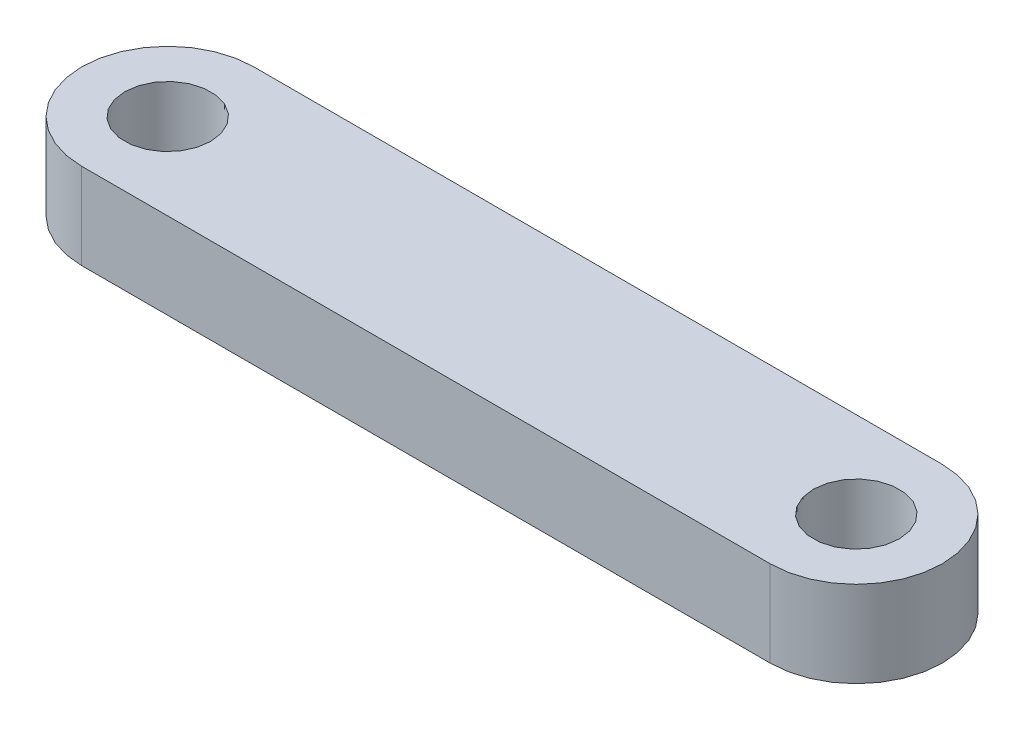
# Autodesk Inventor part: config_arm
Saved by Autodesk Inventor 2021 (Build 250183000, 183)
## iProperties
Created: 2020-12-29
Part Number: config_arm
Material: ABS Plastic
Document SubType Name: Modeling
Designer: Tomasz
Density: 1.06 g/cm^3
Appearance: Smooth - Black
Author: Tomasz
Autodesk Inventor part; units mm, degrees
ref_plane "YZ Plane" through (0, 0, 0) normal (1, 0, 0) x (0, 1, 0)
ref_plane "XZ Plane" through (0, 0, 0) normal (0, 1, 0) x (-1, 0, 0)
ref_plane "XY Plane" through (0, 0, 0) normal (0, 0, 1) x (1, 0, 0)
sketch "Sketch1" plane through (0, 0, 0) normal (0, 1, 0) x (-1, 0, 0)
  line L0 (-4, 0) -> (-36, 0)
  line L1 (-40, -4) -> (-40, -4)
  line L2 (-36, -8) -> (-4, -8)
  line L3 (0, -4) -> (0, -4)
  circle A0 centre (-36, -4) radius 2
  circle A1 centre (-4, -4) radius 2
  arc A2 (-4, -8) -> (0, -4) centre (-4, -4) ccw
  arc A3 (0, -4) -> (-4, 0) centre (-4, -4) ccw
  arc A4 (-36, 0) -> (-40, -4) centre (-36, -4) ccw
  arc A5 (-40, -4) -> (-36, -8) centre (-36, -4) ccw
  point P0 (0, 0)
  point P1 (-40, -8)
  point P2 (-40, 0)
  point P3 (0, -8)
  point P4 (-40, -4)
  point P5 (0, -4)
  dimension "d0" = 40
  dimension "d1" = 8
  dimension "d2" = 4
  dimension "d3" = 4
  dimension "d4" = 4
  dimension "d5" = 4
  dimension "d6" = 4
  dimension "d7" = 4
  dimension "d8" = 4
  constraints: 8 end point, 8 point on circle, 8 point on line, 8 tangent, 6 centre point, 3 equal radius, 2 parallel, 1 horizontal, 1 perpendicular
  measures "d0" distance of point (0, -8) point (-40, -8)
  measures "d1" distance of point (-40, 0) point (-40, -8)
  measures "d2" diameter of A0
  measures "d3" diameter of A1
  measures "d4" distance from line of L1 A0.centre
  measures "d5" distance from line of L2 A0.centre
  measures "d6" distance from line of L3 A1.centre
  measures "d7" distance from line of L2 A1.centre
  measures "d8" radius of A2
extrude "Extrusion1" add sketch "Sketch1" along normal blind 4
equation "\"d1\" = 2 * arm_rod_diam"
equation "\"d2\" = arm_rod_diam"
equation "\"d3\" = arm_rod_diam"
equation "\"d4\" = 0.5 * d1"
equation "\"d5\" = d4"
equation "\"d6\" = d4"
equation "\"d7\" = d5"
equation "\"d8\" = arm_rod_diam"
equation "\"arm_rod_diam\" = 4"
body "Solid1"
